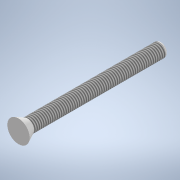
# Autodesk Inventor part: 12_Vite_M3_L30
Saved by Autodesk Inventor 2020 (Build 240168000, 168)
## iProperties
Created: 2019-10-16
Part Number: 12_Vite_M3_L30
Material: Generico
Document SubType Name: Modeling
Designer: socci
Density: 1 g/cm^3
Appearance: Default
Author: socci
Autodesk Inventor part; units mm, degrees
ref_plane "YZ Plane" through (0, 0, 0) normal (1, 0, 0) x (0, 1, 0)
ref_plane "XZ Plane" through (0, 0, 0) normal (0, 1, 0) x (-1, 0, 0)
ref_plane "XY Plane" through (0, 0, 0) normal (0, 0, 1) x (1, 0, 0)
sketch "Schizzo1" plane through (0, 0, 0) normal (0, 1, 0) x (-1, 0, 0)
  line L0 (0, 0) -> (1.5, 0)
  line L1 (0, 0) -> (1.5, 0) construction
  line L2 (0, 2) -> (2.5, 2)
  line L3 (0, 2) -> (2.5, 2) construction
  line L4 (0, 0) -> (0, 2)
  line L5 (2.5, 2) -> (1.5, 0)
  line L6 (1.5, 0) -> (0, 0)
  line L7 (0, 0) -> (0, -30)
  line L8 (0, -30) -> (1.5, -30)
  line L9 (1.5, -30) -> (1.5, 0)
  dimension "d0" = 1.5
  dimension "d2" = 2.5
  dimension "d4" = 2
  dimension "d6" = 30
  constraints: 20 end point, 3 equal length, 3 perpendicular
  measures "d0" distance of L0.start L0.end
  measures "d2" distance of L2.start L2.end
  measures "d4" distance of L0.start L2.start
  measures "d6" distance of L0.start L7.end
revolve "Rivoluzione1" add sketch "Schizzo1" angle 360 about axis through (0, 0, 0) along (0, 0, -1)
fillet "Raccordo1" radius 0.5 1 edges at (1.5, 0, -30)
thread "Filettatura1" size "M3x0.5" class "6g" standard "ANSI Metric M Profile" full length
